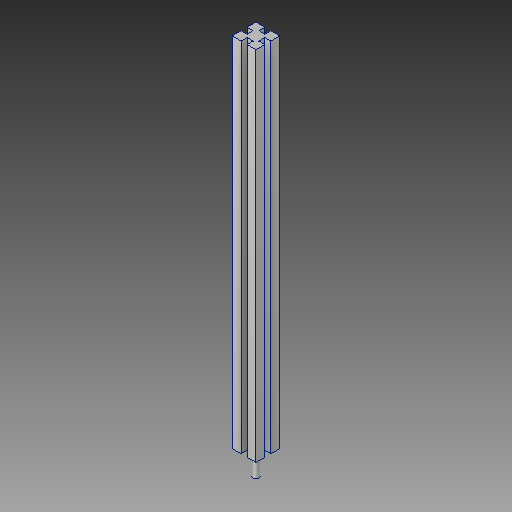
# Autodesk Inventor part: Bauteil2
Saved by Autodesk Inventor 2019 (Build 230136000, 136)
## iProperties
Created: 2021-09-26
Part Number: Bauteil2
Material: Aluminium 6061
Document SubType Name: Modeling
Designer: mritt
Density: 2.7 g/cm^3
Appearance: Aluminium - flach
Author: mritt
Autodesk Inventor part; units mm, degrees
ref_plane "YZ Plane" through (0, 0, 0) normal (1, 0, 0) x (0, 1, 0)
ref_plane "XZ Plane" through (0, 0, 0) normal (0, 1, 0) x (-1, 0, 0)
ref_plane "XY Plane" through (0, 0, 0) normal (0, 0, 1) x (1, 0, 0)
sketch "Skizze1" plane through (0, 0, 0) normal (0, 1, 0) x (-1, 0, 0)
  line L0 (31.1765, -16.3235) -> (11.1765, -16.3235)
  line L1 (11.1765, -16.3235) -> (11.1765, -36.3235)
  line L2 (11.1765, -36.3235) -> (31.1765, -36.3235)
  line L3 (31.1765, -36.3235) -> (31.1765, -16.3235)
  point P0 (0, 0)
  dimension "d0" = 20
  dimension "d1" = 20
  constraints: 8 end point, 2 parallel, 1 horizontal, 1 perpendicular
  measures "d0" distance of L2.end L0.start
  measures "d1" distance of L1.end L2.end
extrude "Extrusion1" add sketch "Skizze1" along normal blind 300
sketch "Skizze2" plane through (0, 0, 0) normal (0, -1, 0) x (1, 0, 0)
  line L0 (-11.1765, -16.3235) -> (-11.1765, -36.3235) projected
  line L1 (-31.1765, -16.3235) -> (-11.1765, -16.3235) projected
  circle A0 centre (-21.1765, -26.3235) radius 2.5676
  point P0 (0, 0)
  dimension "d5" = 10
  dimension "d6" = 10
  constraints: 1 centre point, 1 coincident
  measures "d5" distance from line of point (-21.176, -26.324) L1
  measures "d6" distance from line of point (-21.176, -26.324) L0
extrude "Extrusion2" add sketch "Skizze2" along normal blind 20
sketch "Skizze3" plane through (0, 300, 0) normal (0, 1, 0) x (1, 0, 0)
  line L0 (-11.1765, 16.3235) -> (-11.1765, 36.3235) projected
  line L1 (-11.1765, 23.8235) -> (-16.1765, 23.8235)
  line L2 (-16.1765, 23.8235) -> (-16.1765, 28.8235)
  line L3 (-16.1765, 28.8235) -> (-11.1765, 28.8235)
  line L4 (-11.1765, 28.8235) -> (-11.1765, 23.8235)
  line L5 (-11.1765, 36.3235) -> (-31.1765, 36.3235) projected
  line L6 (-23.6765, 36.3235) -> (-18.6765, 36.3235)
  line L7 (-18.6765, 36.3235) -> (-18.6765, 31.3235)
  line L8 (-18.6765, 31.3235) -> (-23.6765, 31.3235)
  line L9 (-23.6765, 31.3235) -> (-23.6765, 36.3235)
  line L10 (-31.1765, 23.8235) -> (-26.1765, 23.8235)
  line L11 (-26.1765, 23.8235) -> (-26.1765, 28.8235)
  line L12 (-26.1765, 28.8235) -> (-31.1765, 28.8235)
  line L13 (-31.1765, 28.8235) -> (-31.1765, 23.8235)
  line L14 (-31.1765, 16.3235) -> (-11.1765, 16.3235) projected
  line L15 (-23.6765, 16.3235) -> (-18.6765, 16.3235)
  line L16 (-18.6765, 16.3235) -> (-18.6765, 21.3235)
  line L17 (-18.6765, 21.3235) -> (-23.6765, 21.3235)
  line L18 (-23.6765, 21.3235) -> (-23.6765, 16.3235)
  line L19 (-31.1765, 36.3235) -> (-31.1765, 16.3235) projected
  point P0 (0, 0)
  dimension "d9" = 5
  dimension "d10" = 7.5
  dimension "d11" = 7.5
  dimension "d12" = 5
  dimension "d13" = 7.5
  dimension "d14" = 5
  dimension "d15" = 5
  dimension "d16" = 7.5
  dimension "d17" = 5
  dimension "d18" = 5
  dimension "d19" = 5
  dimension "d20" = 5
  constraints: 32 end point, 8 parallel, 4 horizontal, 4 perpendicular, 3 point on line, 1 collinear
  measures "d9" distance of L7.end L8.end
  measures "d10" distance from line of L8.end L19
  measures "d11" distance between parallel lines of L1 L14
  measures "d12" distance of L1.end L2.end
  measures "d13" distance between parallel lines of L18 L19
  measures "d14" distance of L16.end L17.end
  measures "d15" distance of L10.end L11.end
  measures "d16" distance between parallel lines of L10 L14
  measures "d17" distance of L11.end L12.end
  measures "d18" distance of L6.end L7.end
  measures "d19" distance of L2.end L3.end
  measures "d20" distance of L15.end L16.end
extrude "Extrusion3" cut sketch "Skizze3" against normal blind 300 contours L1 L2 L3 L0 | L14 L18 L17 L16 | L7 L8 L9 L5 | L13 L12 L11 L10
